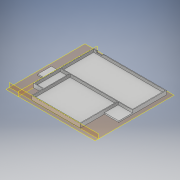
# Autodesk Inventor part: Entrance_System
Saved by Autodesk Inventor 2019 (Build 230136000, 136)
## iProperties
Created: 2019-10-13
Part Number: Entrance_System
Material: Všeobecné
Document SubType Name: Modeling
Designer: Barsonica
Density: 1 g/cm^3
Appearance: Výchozí
Author: Barsonica
Autodesk Inventor part; units mm, degrees
sketch "Náčrt1" plane through (0, 0, 0) normal (0, 1, 0) x (-1, 0, 0)
  line L0 (0, 0) -> (-86, 0)
  line L1 (-86, 0) -> (-86, -55.5)
  line L2 (-86, -55.5) -> (0, -55.5)
  line L3 (0, -55.5) -> (0, 0)
  line L4 (0, -55.5) -> (0, -105.5)
  line L5 (0, -105.5) -> (-107, -105.5)
  line L6 (-107, -105.5) -> (-107, -55.5)
  line L7 (-107, -55.5) -> (-86, -55.5)
  dimension "d0" = 86
  dimension "d1" = 55.5
  dimension "d2" = 90
  dimension "d3" = 50
  dimension "d4" = 107
  constraints: 16 end point, 6 perpendicular, 2 point on line, 1 horizontal
  measures "d0" distance of L0.start L0.end
  measures "d1" distance of L0.end L1.end
  measures "d2" angle of L1 L0
  measures "d3" distance of L2.end L4.end
  measures "d4" distance of L4.end L5.end
extrude "Vysunutí1" add sketch "Náčrt1" along normal blind 1.8
sketch "Náčrt2" plane through (0, 1.8, 0) normal (0, 1, 0) x (1, 0, 0)
  line L0 (107, 105.5) -> (0, 105.5) projected
  line L1 (107, 55.5) -> (107, 105.5) projected
  line L2 (86, 55.5) -> (107, 55.5) projected
  line L3 (86, 0) -> (86, 55.5) projected
  line L4 (0, 0) -> (86, 0) projected
  line L5 (0, 105.5) -> (0, 0) projected
  line L6 (85, 1) -> (85, 55.5)
  line L7 (14.5, 55.5) -> (14.5, 0)
  line L8 (15.5, 55.5) -> (85, 55.5)
  line L9 (1, 56.5) -> (106, 56.5)
  line L10 (1, 56.5) -> (1, 104.5)
  line L11 (1, 104.5) -> (106, 104.5)
  line L12 (106, 104.5) -> (106, 56.5)
  line L13 (15.5, 1) -> (85, 1)
  line L14 (15.5, 55.5) -> (15.5, 1)
  line L15 (14.5, 55.5) -> (1, 55.5)
  line L16 (1, 55.5) -> (1, 18)
  line L17 (1, 18) -> (14.5, 18)
  line L18 (0, 17) -> (14.5, 17)
  dimension "d21" = 14.5
  dimension "d22" = 1
  dimension "d23" = 1
  dimension "d24" = 48
  dimension "d25" = 105
  dimension "d28" = 1
  dimension "d29" = 37.5
  dimension "d30" = 1
  dimension "d31" = 1
  dimension "d45" = 1
  dimension "d46" = 1
  dimension "d47" = 1
  dimension "d48" = 54.5
  dimension "d49" = 1
  dimension "d50" = 1
  dimension "d51" = 69.5
  constraints: 26 end point, 6 perpendicular, 4 point on line, 3 horizontal, 2 parallel, 1 vertical
  measures "d21" distance between parallel lines of L5 L7
  measures "d22" distance from line of L5 L9.start
  measures "d23" distance from line of L1 L9.end
  measures "d24" distance of L9.start L10.end
  measures "d25" distance of L10.end L11.end
  measures "d28" distance between parallel lines of L8 L9
  measures "d29" distance of L15.end L16.end
  measures "d30" distance between parallel lines of L5 L16
  measures "d31" distance between parallel lines of L17 L18
  measures "d45" distance between parallel lines of L0 L11
  measures "d46" distance between parallel lines of L3 L6
  measures "d47" distance between parallel lines of L4 L13
  measures "d48" distance between parallel lines of L13 L8
  measures "d49" distance between parallel lines of L9 L15
  measures "d50" distance between parallel lines of L14 L7
  measures "d51" distance between parallel lines of L6 L14
extrude "Vysunutí3" add sketch "Náčrt2" along normal blind 4 contours L1 L2 L3 L4 L7 L18 L5 L0
sketch "Náčrt3" plane through (0, 1.8, 0) normal (0, 1, 0) x (1, 0, 0)
  line L0 (14.5, 17) -> (0, 17) projected
  line L1 (0, 17) -> (0, 0) projected
  line L2 (0, 0) -> (14.5, 0) projected
  line L3 (14.5, 0) -> (14.5, 17) projected
extrude "Vysunutí4" cut sketch "Náčrt3" against normal blind 4
sketch "Náčrt4" plane through (107, 0, -105.5) normal (0, 0, -1) x (-1, 0, 0)
  line L0 (101, 3.2) -> (94, 3.2)
  line L1 (101, 3.2) -> (101, 5.8)
  line L2 (101, 3.2) -> (103.6, 3.2) construction
  line L3 (94, 5.8) -> (94, 3.2)
  line L4 (0, 5.8) -> (107, 5.8) projected
  line L5 (107, 0) -> (107, 5.8) projected
  line L6 (106, 5.8) -> (92.5, 5.8) projected
  line L7 (101, 5.8) -> (92.5, 5.8)
  dimension "d37" = 7
  dimension "d39" = 90
  dimension "d41" = 6
  dimension "d42" = 3.6
  constraints: 10 end point, 3 perpendicular, 2 horizontal, 2 point on line, 1 collinear, 1 vertical
  measures "d37" distance of L0.start L0.end
  measures "d39" angle of L2 L1
  measures "d41" distance between parallel lines of L5 L1
sketch "Náčrt4 outline for Vysunutí5" plane through (107, 0, -105.5) normal (0, 0, -1) x (-1, 0, 0)
  line L0 (94, 3.2) -> (101, 3.2)
  line L1 (92.5, 5.8) -> (94, 3.2)
  line L2 (101, 5.8) -> (92.5, 5.8)
  line L3 (101, 3.2) -> (101, 5.8)
extrude "Vysunutí5" cut sketch "Náčrt4 outline for Vysunutí5" against normal blind 4
sketch "Sketch5" plane through (0, 0, 0) normal (0, 1, 0) x (-1, 0, 0)
  line L0 (-86, -55.5) -> (-107, -55.5) projected
  line L1 (-107, -55.5) -> (-107, -35.5)
  line L2 (-107, -35.5) -> (-86, -35.5)
  line L3 (-86, 0) -> (-86, -55.5) projected
  line L4 (0, -105.5) -> (0, -17) projected
  line L5 (0, -55.5) -> (12, -55.5)
  line L6 (12, -55.5) -> (12, -35.5)
  line L7 (12, -35.5) -> (0, -35.5)
  line L8 (0, -35.5) -> (0, -55.5)
  line L9 (-1, -55.5) -> (-14.5, -55.5) projected
  line L10 (0, -17) -> (-14.5, -17) projected
  point P0 (0, 0)
  dimension "d52" = 20
  dimension "d53" = 12
  dimension "d54" = 20
  dimension "d55" = 18.5
  constraints: 12 end point, 2 parallel, 2 perpendicular, 2 point on line, 1 collinear, 1 horizontal, 1 vertical
  measures "d52" distance of L0.end L1.end
  measures "d53" distance of L7.end L6.end
  measures "d54" distance of L6.end L5.end
  measures "d55" distance from line of L10 L7.end
extrude "Extrusion6" add sketch "Sketch5" along normal blind 2
